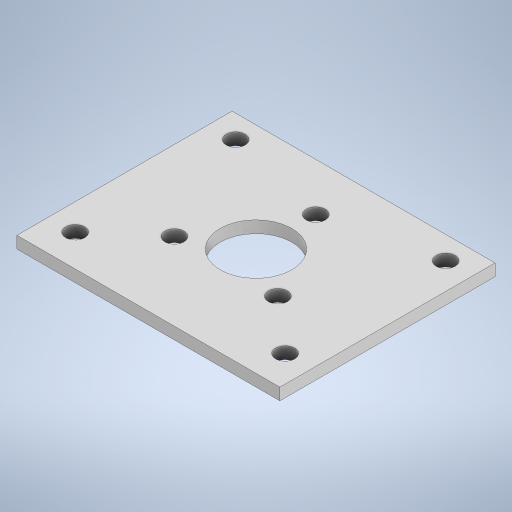
# Autodesk Inventor part: motorbracket2
Saved by Autodesk Inventor 2024.3 (Build 283343000, 343)
## iProperties
Created: 2024-11-20
Part Number: motorbracket2
Material: Generic
Document SubType Name: Modeling
Designer: email
Density: 1 g/cm^3
Appearance: Default
Author: email
Autodesk Inventor part; units mm, degrees
ref_plane "YZ Plane" through (0, 0, 0) normal (1, 0, 0) x (0, 1, 0)
ref_plane "XZ Plane" through (0, 0, 0) normal (0, 1, 0) x (-1, 0, 0)
ref_plane "XY Plane" through (0, 0, 0) normal (0, 0, 1) x (1, 0, 0)
sketch "Sketch1" plane through (0, 0, 0) normal (0, 1, 0) x (-1, 0, 0)
  line L0 (0, 0) -> (-110, 0)
  line L1 (-110, 0) -> (-110, -90)
  line L2 (-110, -90) -> (0, -90)
  line L3 (0, -90) -> (0, 0)
  line L4 (0, -90) -> (-11.075, -90)
  line L5 (-11.075, -90) -> (-11.075, 0) construction
  line L6 (-11.075, 0) -> (0, 0)
  line L7 (0, 0) -> (0, -90)
  line L8 (-110, -90) -> (-98.925, -90)
  line L9 (-98.925, -90) -> (-98.925, 0) construction
  line L10 (-98.925, 0) -> (-110, 0)
  line L11 (-110, 0) -> (-110, -90)
  line L12 (-11.075, -90) -> (-11.075, -84)
  circle A0 centre (-11.075, -80.425) radius 3.575
  line L13 (-11.075, -76.85) -> (-11.075, -16.85) construction
  circle A1 centre (-11.075, -13.275) radius 3.575
  line L14 (-98.925, -90) -> (-98.925, -84)
  circle A2 centre (-98.925, -80.425) radius 3.575
  line L15 (-98.925, -76.85) -> (-98.925, -16.85) construction
  circle A3 centre (-98.925, -13.275) radius 3.575
  line L16 (-55, 0) -> (-55, -45)
  circle A4 centre (-55, -45) radius 15
  circle A5 centre (-55, -45) radius 25
  circle A6 centre (-55, -70) radius 3.25
  circle A7 centre (-33.3494, -32.5) radius 3.25
  circle A8 centre (-76.6506, -32.5) radius 3.25
  dimension "d7" = 7.15
  dimension "d11" = 7.15
  dimension "d15" = 50
  dimension "d0" = 90
  dimension "d1" = 110
  dimension "d2" = 11.075
  dimension "d3" = 11.075
  dimension "d4" = 6
  dimension "d5" = 7.15
  dimension "d6" = 60
  dimension "d8" = 6
  dimension "d9" = 7.15
  dimension "d10" = 60
  dimension "d12" = 55
  dimension "d13" = 45
  dimension "d14" = 30
  dimension "d16" = 6.5
  dimension "d19" = 360
  dimension "d37" = 87.85
  constraints: 34 end point, 12 point on line, 6 centre point, 6 parallel, 4 point on circle, 3 horizontal, 3 perpendicular, 3 vertical alignment, 2 coincident, 1 midpoint, 1 vertical, 13 other
  measures "d0" distance of L0.end L1.end
  measures "d1" distance of L1.end L2.end
  measures "d2" distance between parallel lines of L3 L5
  measures "d3" distance between parallel lines of L1 L9
  measures "d4" distance of L4.end L12.end
  measures "d5" diameter of A0
  measures "d6" distance of L13.start L13.end
  measures "d8" distance of L8.end L14.end
  measures "d9" diameter of A2
  measures "d10" distance of L15.start L15.end
  measures "d12" distance between parallel lines of L3 L16
  measures "d13" distance of L16.start L16.end
  measures "d14" diameter of A4
  measures "d16" diameter of A6
  measures "d37" distance of point (-11.075, -13.275) point (-98.925, -13.275)
extrude "Extrusion1" add sketch "Sketch1" along normal blind 5 contours A5 A7 A6 A8 | A2 | A0 | L3 L2 L1 L0 | A7 A5 | A5 A7 | A8 A5 | A5 A8 | A6 A5 | A5 A6 | A1 | A3
hole "Hole1" at (98.925, 0, -80.425) at (11.075, 0, -80.425) at (11.075, 0, -13.275) at (98.925, 0, -13.275) direction (0, 1, 0) diameter 8 depth 10
hole "Hole2" at (55, 0, -70) at (76.6506, 0, -32.5) at (33.3494, 0, -32.5) direction (0, 1, 0) diameter 8 depth 10
body "Solid1"
